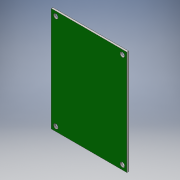
# Autodesk Inventor part: regulator
Saved by Autodesk Inventor 2016 (Build 200138000, 138)
## iProperties
Created: 2016-09-22
Part Number: regulator
Material: Generic
Document SubType Name: Modeling
Designer: Jakub
Density: 1 g/cm^3
Appearance: Default
Mass: 2.41637 g
Surface Area: 50.6415 cm^2
Volume: 2.41637 cm^3
Author: Jakub
Autodesk Inventor part; units mm, degrees
ref_plane "YZ Plane" through (0, 0, 0) normal (1, 0, 0) x (0, 1, 0)
ref_plane "XZ Plane" through (0, 0, 0) normal (0, 1, 0) x (-1, 0, 0)
ref_plane "XY Plane" through (0, 0, 0) normal (0, 0, 1) x (1, 0, 0)
sketch "Sketch1" plane through (0, 0, 0) normal (0, 1, 0) x (-1, 0, 0)
  line L0 (-21, 29) -> (21, 29)
  line L1 (21, 29) -> (21, -29)
  line L2 (21, -29) -> (-21, -29)
  line L3 (-21, -29) -> (-21, 29)
  line L4 (-21, 29) -> (21, -29) construction
  line L5 (21, 29) -> (-21, -29) construction
  point P0 (0, 0)
  dimension "d0" = 42
  dimension "d1" = 58
  constraints: 12 end point, 2 midpoint, 2 parallel, 1 horizontal, 1 perpendicular
  measures "d0" distance of L1.end L2.end
  measures "d1" distance of L0.end L1.end
extrude "Extrusion1" add sketch "Sketch1" along normal blind 1
sketch "Sketch2" plane through (0, 1, 0) normal (0, 1, 0) x (1, 0, 0)
  line L0 (-20.998, 28.8101) -> (20.8952, 28.8101) construction
  line L1 (20.8952, 28.8101) -> (20.8952, -28.9985) construction
  line L2 (20.8952, -28.9985) -> (-20.998, -28.9985) construction
  line L3 (-20.998, -28.9985) -> (-20.998, 28.8101) construction
  point P0 (0, 0)
  constraints: 2 other
sketch "Sketch3" plane through (0, 0, 0) normal (0, -1, 0) x (1, 0, 0)
  line L0 (-20.9976, 28.7529) -> (21.0508, 28.7529) construction
  line L1 (21.0508, 28.7529) -> (21.0508, -28.9972) construction
  line L2 (21.0508, -28.9972) -> (-20.9976, -28.9972) construction
  line L3 (-20.9976, -28.9972) -> (-20.9976, 28.7529) construction
  point P0 (0, 0)
  constraints: 2 other
sketch "Sketch4" plane through (0, 0, 0) normal (0, -1, 0) x (1, 0, 0)
  line L0 (-21, 29) -> (21, 29) projected
  line L1 (21, 29) -> (18.5, 29)
  line L2 (18.5, 29) -> (18.5, 26.5)
  line L3 (18.5, 26.5) -> (21, 26.5)
  line L4 (21, 26.5) -> (21, 29)
  circle A0 centre (18.5, 26.5) radius 1.25
  point P0 (0, 0)
  dimension "d42" = 2.5
  dimension "d43" = 2.5
  dimension "d44" = 2.5
  constraints: 8 end point, 2 parallel, 1 centre point, 1 coincident, 1 horizontal, 1 perpendicular
  measures "d42" distance of L3.end L2.end
  measures "d43" distance of L2.end L1.end
  measures "d44" diameter of A0
extrude "Extrusion2" cut sketch "Sketch4" against normal through all contours A0 L3 L2 | L2 L3 A0
sketch "Sketch5" plane through (0, 0, 0) normal (0, -1, 0) x (1, 0, 0)
  line L0 (-21, -29) -> (21, -29) projected
  line L1 (-21, -29) -> (-18.5, -29)
  line L2 (-18.5, -29) -> (-18.5, -26.5)
  line L3 (-18.5, -26.5) -> (-21, -26.5)
  line L4 (-21, -26.5) -> (-21, -29)
  circle A0 centre (-18.5, -26.5) radius 1.25
  point P0 (0, 0)
  dimension "d49" = 2.5
  dimension "d50" = 2.5
  dimension "d51" = 2.5
  constraints: 8 end point, 2 parallel, 1 centre point, 1 coincident, 1 horizontal, 1 perpendicular
  measures "d49" distance of L3.end L2.end
  measures "d50" distance of L2.end L1.end
  measures "d51" diameter of A0
extrude "Extrusion3" cut sketch "Sketch5" against normal through all contours A0 L3 L2 | L2 L3 A0
sketch "Sketch6" plane through (0, 1, 0) normal (0, 1, 0) x (1, 0, 0)
  line L0 (-21, -29) -> (21, -29) projected
  line L1 (-21, -29) -> (-18.5, -29)
  line L2 (-18.5, -29) -> (-18.5, -26.5)
  line L3 (-18.5, -26.5) -> (-21, -26.5)
  line L4 (-21, -26.5) -> (-21, -29)
  circle A0 centre (-18.5, -26.5) radius 1.25
  point P0 (0, 0)
  dimension "d60" = 2.5
  dimension "d61" = 2.5
  dimension "d62" = 2.5
  constraints: 8 end point, 2 parallel, 1 centre point, 1 coincident, 1 horizontal, 1 perpendicular
  measures "d60" distance of L3.end L2.end
  measures "d61" distance of L2.end L1.end
  measures "d62" diameter of A0
extrude "Extrusion4" cut sketch "Sketch6" against normal up to next contours A0 L3 L2 | L2 L3 A0
sketch "Sketch7" plane through (0, 0, 0) normal (0, -1, 0) x (1, 0, 0)
  circle A0 centre (18.5, -26.5) radius 1.25
  line L0 (-21, -29) -> (21, -29) projected
  line L1 (21, -29) -> (21, 29) projected
  point P0 (0, 0)
  dimension "d67" = 2.5
  dimension "d68" = 2.5
  dimension "d69" = 2.5
  constraints: 1 centre point
  measures "d67" diameter of A0
  measures "d68" distance from line of L0 A0.centre
  measures "d69" distance from line of L1 A0.centre
extrude "Extrusion5" cut sketch "Sketch7" against normal up to next
body "Solid1"
